Autodesk Fusion 360 part; units mm, degrees
(part 2 of 3)
  spline S228 degree 3 poles (-3.1149, 116.9539) (-3.0452, 117.0404) (-2.9015, 117.2184) (-2.6994, 117.3259) (-2.5954, 117.3812) knots 0 0 0 0 0.032959 0.067885 0.067885 0.067885 0.067885
  spline S229 degree 3 poles (-3.3935, 116.2276) (-3.362, 116.3667) (-3.304, 116.6225) (-3.1742, 116.8501) (-3.1149, 116.9539) knots 0 0 0 0 0.042495 0.07817 0.07817 0.07817 0.07817
  line L121 (-3.3935, 116.2276) -> (-2.5083, 116.0772)
  spline S230 degree 3 poles (-2.2963, 116.5763) (-2.3491, 116.5089) (-2.4641, 116.3621) (-2.4927, 116.1772) (-2.5083, 116.0772) knots 0 0 0 0 0.025264 0.055024 0.055024 0.055024 0.055024
  spline S231 degree 3 poles (-1.8759, 116.7471) (-1.9549, 116.7401) (-2.1125, 116.726) (-2.2351, 116.6261) (-2.2963, 116.5763) knots 0 0 0 0 0.023212 0.046318 0.046318 0.046318 0.046318
  spline S232 degree 3 poles (-1.476, 116.5968) (-1.532, 116.6406) (-1.6492, 116.7324) (-1.7981, 116.7421) (-1.8759, 116.7471) knots 0 0 0 0 0.020834 0.04362 0.04362 0.04362 0.04362
  spline S233 degree 3 poles (-1.3256, 116.1934) (-1.3306, 116.2721) (-1.34, 116.4222) (-1.4322, 116.5405) (-1.476, 116.5968) knots 0 0 0 0 0.023038 0.043945 0.043945 0.043945 0.043945
  spline S234 degree 3 poles (-1.5307, 115.7166) (-1.4709, 115.7825) (-1.3482, 115.9178) (-1.3333, 116.1) (-1.3256, 116.1934) knots 0 0 0 0 0.025943 0.053218 0.053218 0.053218 0.053218
  spline S235 degree 3 poles (-2.1254, 115.5474) (-2.0075, 115.5485) (-1.7927, 115.5505) (-1.6121, 115.665) (-1.5307, 115.7166) knots 0 0 0 0 0.034551 0.062931 0.062931 0.062931 0.062931
  line L122 (-2.1254, 115.5474) -> (-2.2314, 114.7647)
  spline S236 degree 3 poles (-1.7905, 114.8365) (-1.8583, 114.8326) (-2.0077, 114.8239) (-2.1524, 114.7856) (-2.2314, 114.7647) knots 0 0 0 0 0.020331 0.044771 0.044771 0.044771 0.044771
  spline S237 degree 3 poles (-1.3154, 114.6246) (-1.3835, 114.6864) (-1.5188, 114.8091) (-1.7004, 114.8274) (-1.7905, 114.8365) knots 0 0 0 0 0.026832 0.05326 0.05326 0.05326 0.05326
  spline S238 degree 3 poles (-1.1206, 114.0504) (-1.1264, 114.1623) (-1.1374, 114.3727) (-1.2586, 114.5443) (-1.3154, 114.6246) knots 0 0 0 0 0.032834 0.061749 0.061749 0.061749 0.061749
  spline S239 degree 3 poles (-1.3239, 113.442) (-1.2647, 113.5273) (-1.1381, 113.7097) (-1.1267, 113.9321) (-1.1206, 114.0504) knots 0 0 0 0 0.030567 0.065292 0.065292 0.065292 0.065292
  spline S240 degree 3 poles (-1.8247, 113.2164) (-1.7293, 113.226) (-1.5373, 113.2454) (-1.3953, 113.3762) (-1.3239, 113.442) knots 0 0 0 0 0.027961 0.056262 0.056262 0.056262 0.056262
  spline S241 degree 3 poles (-2.2963, 113.4044) (-2.2277, 113.3495) (-2.0895, 113.2392) (-1.9133, 113.224) (-1.8247, 113.2164) knots 0 0 0 0 0.025738 0.0518 0.0518 0.0518 0.0518
  spline S242 degree 3 poles (-2.5356, 113.9478) (-2.5173, 113.8392) (-2.4833, 113.6372) (-2.3554, 113.4779) (-2.2963, 113.4044) knots 0 0 0 0 0.032415 0.060264 0.060264 0.060264 0.060264
  line L123 (-2.5356, 113.9478) -> (-3.4653, 113.835)
  spline S243 degree 3 poles (-2.9458, 112.8114) (-3.0795, 112.9538) (-3.3522, 113.244) (-3.4271, 113.6356) (-3.4653, 113.835) knots 0 0 0 0 0.057366 0.116928 0.116928 0.116928 0.116928
  line L124 (-5.3383, 113.2266) -> (-5.3383, 114.5289)
  line L125 (-5.3383, 114.5289) -> (-4.0224, 114.5289)
  line L126 (-4.0224, 114.5289) -> (-4.0224, 115.4278)
  line L127 (-4.0224, 115.4278) -> (-5.3383, 115.4278)
  line L128 (-5.3383, 115.4278) -> (-5.3383, 116.7301)
  line L129 (-5.3383, 116.7301) -> (-6.2133, 116.7301)
  line L130 (-6.2133, 116.7301) -> (-6.2133, 115.4278)
  line L131 (-6.2133, 115.4278) -> (-7.5258, 115.4278)
  line L132 (-7.5258, 115.4278) -> (-7.5258, 114.5289)
  line L133 (-7.5258, 114.5289) -> (-6.2133, 114.5289)
  line L134 (-6.2133, 114.5289) -> (-6.2133, 113.2266)
  line L135 (-6.2133, 113.2266) -> (-5.3383, 113.2266)
  line L136 (20.9668, 130.42) -> (22.8707, 130.42)
  spline S244 degree 3 poles (23.7662, 130.526) (23.6363, 130.4952) (23.3421, 130.4254) (23.0396, 130.4219) (22.8707, 130.42) knots 0 0 0 0 0.039934 0.090419 0.090419 0.090419 0.090419
  spline S245 degree 3 poles (24.4771, 130.9259) (24.3774, 130.8438) (24.1645, 130.6685) (23.9045, 130.5754) (23.7662, 130.526) knots 0 0 0 0 0.038436 0.082116 0.082116 0.082116 0.082116
  spline S246 degree 3 poles (25.0137, 131.8111) (24.9472, 131.6403) (24.82, 131.3136) (24.5879, 131.0511) (24.4771, 130.9259) knots 0 0 0 0 0.054482 0.104246 0.104246 0.104246 0.104246
  spline S247 degree 3 poles (25.1675, 132.8775) (25.1631, 132.6843) (25.1547, 132.3224) (25.0585, 131.9737) (25.0137, 131.8111) knots 0 0 0 0 0.057721 0.108107 0.108107 0.108107 0.108107
  spline S248 degree 3 poles (25.0035, 134.0618) (25.0512, 133.8841) (25.1554, 133.4965) (25.1633, 133.0949) (25.1675, 132.8775) knots 0 0 0 0 0.055013 0.119956 0.119956 0.119956 0.119956
  spline S249 degree 3 poles (24.525, 134.8736) (24.6242, 134.7548) (24.8282, 134.5107) (24.944, 134.2141) (25.0035, 134.0618) knots 0 0 0 0 0.046108 0.094787 0.094787 0.094787 0.094787
  spline S250 degree 3 poles (23.7696, 135.335) (23.9112, 135.2834) (24.194, 135.1804) (24.4148, 134.9758) (24.525, 134.8736) knots 0 0 0 0 0.044725 0.089312 0.089312 0.089312 0.089312
  spline S251 degree 3 poles (22.816, 135.4307) (23.0005, 135.4297) (23.3217, 135.428) (23.6358, 135.3628) (23.7696, 135.335) knots 0 0 0 0 0.055167 0.096048 0.096048 0.096048 0.096048
  line L137 (22.816, 135.4307) -> (20.9668, 135.4307)
  line L138 (20.9668, 135.4307) -> (20.9668, 130.42)
  spline S252 degree 3 poles (23.2637, 134.5352) (23.1593, 134.549) (22.8839, 134.5853) (22.6058, 134.5839) (22.4332, 134.5831) knots 0 0 0 0 0.031565 0.083275 0.083275 0.083275 0.083275
  spline S253 degree 3 poles (23.732, 134.2994) (23.6648, 134.3531) (23.5254, 134.4645) (23.353, 134.5111) (23.2637, 134.5352) knots 0 0 0 0 0.02553 0.052932 0.052932 0.052932 0.052932
  spline S254 degree 3 poles (24.0191, 133.814) (23.9838, 133.9098) (23.9176, 134.0893) (23.7911, 134.2325) (23.732, 134.2994) knots 0 0 0 0 0.030297 0.056827 0.056827 0.056827 0.056827
  spline S255 degree 3 poles (24.1216, 132.922) (24.1204, 133.0941) (24.1182, 133.3954) (24.0488, 133.6884) (24.0191, 133.814) knots 0 0 0 0 0.051419 0.090046 0.090046 0.090046 0.090046
  spline S256 degree 3 poles (24.0191, 132.0042) (24.0489, 132.1363) (24.1169, 132.4381) (24.1199, 132.7478) (24.1216, 132.922) knots 0 0 0 0 0.040513 0.092572 0.092572 0.092572 0.092572
  spline S257 degree 3 poles (23.7542, 131.5206) (23.8074, 131.5831) (23.9287, 131.7255) (23.9866, 131.904) (24.0191, 132.0042) knots 0 0 0 0 0.024396 0.055616 0.055616 0.055616 0.055616
  spline S258 degree 3 poles (23.3458, 131.3121) (23.4232, 131.3352) (23.5723, 131.3796) (23.6951, 131.4748) (23.7542, 131.5206) knots 0 0 0 0 0.023993 0.046213 0.046213 0.046213 0.046213
  spline S259 degree 3 poles (22.7339, 131.2642) (22.8559, 131.2642) (23.0613, 131.2642) (23.2636, 131.2983) (23.3458, 131.3121) knots 0 0 0 0 0.036506 0.061461 0.061461 0.061461 0.061461
  line L139 (22.7339, 131.2642) -> (21.9786, 131.2642)
  line L140 (21.9786, 131.2642) -> (21.9786, 134.5831)
  line L141 (21.9786, 134.5831) -> (22.4332, 134.5831)
  line L142 (26.9517, 130.42) -> (26.9517, 134.3643)
  line L143 (26.9517, 134.3643) -> (27.9429, 130.42)
  line L144 (27.9429, 130.42) -> (28.917, 130.42)
  line L145 (28.917, 130.42) -> (29.9117, 134.3643)
  line L146 (29.9117, 134.3643) -> (29.9117, 130.42)
  line L147 (29.9117, 130.42) -> (30.8516, 130.42)
  line L148 (30.8516, 130.42) -> (30.8516, 135.4307)
  line L149 (30.8516, 135.4307) -> (29.334, 135.4307)
  line L150 (29.334, 135.4307) -> (28.4351, 132.0128)
  line L151 (28.4351, 132.0128) -> (27.5259, 135.4307)
  line L152 (27.5259, 135.4307) -> (26.0118, 135.4307)
  line L153 (26.0118, 135.4307) -> (26.0118, 130.42)
  line L154 (26.0118, 130.42) -> (26.9517, 130.42)
  line L155 (32.7828, 130.42) -> (32.7828, 134.3643)
  line L156 (32.7828, 134.3643) -> (33.774, 130.42)
  line L157 (33.774, 130.42) -> (34.7481, 130.42)
  line L158 (34.7481, 130.42) -> (35.7427, 134.3643)
  line L159 (35.7427, 134.3643) -> (35.7427, 130.42)
  line L160 (35.7427, 130.42) -> (36.6827, 130.42)
  line L161 (36.6827, 130.42) -> (36.6827, 135.4307)
  line L162 (36.6827, 135.4307) -> (35.1651, 135.4307)
  line L163 (35.1651, 135.4307) -> (34.2662, 132.0128)
  line L164 (34.2662, 132.0128) -> (33.357, 135.4307)
  line L165 (33.357, 135.4307) -> (31.8428, 135.4307)
  line L166 (31.8428, 135.4307) -> (31.8428, 130.42)
  line L167 (31.8428, 130.42) -> (32.7828, 130.42)
  line L168 (39.9332, 135.4513) -> (39.1539, 135.4513)
  spline S260 degree 3 poles (38.5489, 134.6497) (38.6832, 134.766) (38.9423, 134.9903) (39.0851, 135.3014) (39.1539, 135.4513) knots 0 0 0 0 0.052597 0.101463 0.101463 0.101463 0.101463
  spline S261 degree 3 poles (37.732, 134.1832) (37.8654, 134.2377) (38.1579, 134.3572) (38.4112, 134.5467) (38.5489, 134.6497) knots 0 0 0 0 0.043078 0.094413 0.094413 0.094413 0.094413
  line L169 (37.732, 134.1832) -> (37.732, 133.3116)
  spline S262 degree 3 poles (38.9727, 134.0396) (38.7881, 133.8858) (38.4148, 133.5747) (37.9613, 133.4) (37.732, 133.3116) knots 0 0 0 0 0.071555 0.144721 0.144721 0.144721 0.144721
  line L170 (38.9727, 134.0396) -> (38.9727, 130.42)
  line L171 (38.9727, 130.42) -> (39.9332, 130.42)
  line L172 (39.9332, 130.42) -> (39.9332, 135.4513)
  line L173 (20.5738, 112.42) -> (22.4776, 112.42)
  spline S263 degree 3 poles (23.3731, 112.526) (23.2432, 112.4952) (22.9491, 112.4254) (22.6465, 112.4219) (22.4776, 112.42) knots 0 0 0 0 0.039934 0.090419 0.090419 0.090419 0.090419
  spline S264 degree 3 poles (24.084, 112.9259) (23.9844, 112.8438) (23.7714, 112.6685) (23.5114, 112.5754) (23.3731, 112.526) knots 0 0 0 0 0.038436 0.082116 0.082116 0.082116 0.082116
  spline S265 degree 3 poles (24.6207, 113.8111) (24.5541, 113.6403) (24.4269, 113.3136) (24.1948, 113.0511) (24.084, 112.9259) knots 0 0 0 0 0.054482 0.104246 0.104246 0.104246 0.104246
  spline S266 degree 3 poles (24.7745, 114.8775) (24.77, 114.6843) (24.7616, 114.3224) (24.6655, 113.9737) (24.6207, 113.8111) knots 0 0 0 0 0.057721 0.108107 0.108107 0.108107 0.108107
  spline S267 degree 3 poles (24.6104, 116.0618) (24.6582, 115.8841) (24.7623, 115.4965) (24.7702, 115.0949) (24.7745, 114.8775) knots 0 0 0 0 0.055013 0.119956 0.119956 0.119956 0.119956
  spline S268 degree 3 poles (24.1319, 116.8736) (24.2311, 116.7548) (24.4352, 116.5107) (24.5509, 116.2141) (24.6104, 116.0618) knots 0 0 0 0 0.046108 0.094787 0.094787 0.094787 0.094787
  spline S269 degree 3 poles (23.3765, 117.335) (23.5181, 117.2834) (23.8009, 117.1804) (24.0217, 116.9758) (24.1319, 116.8736) knots 0 0 0 0 0.044725 0.089312 0.089312 0.089312 0.089312
  spline S270 degree 3 poles (22.4229, 117.4307) (22.6074, 117.4297) (22.9286, 117.428) (23.2428, 117.3628) (23.3765, 117.335) knots 0 0 0 0 0.055167 0.096048 0.096048 0.096048 0.096048
  line L174 (22.4229, 117.4307) -> (20.5738, 117.4307)
  line L175 (20.5738, 117.4307) -> (20.5738, 112.42)
  spline S271 degree 3 poles (22.8707, 116.5352) (22.7662, 116.549) (22.4908, 116.5853) (22.2127, 116.5839) (22.0401, 116.5831) knots 0 0 0 0 0.031565 0.083275 0.083275 0.083275 0.083275
  spline S272 degree 3 poles (23.3389, 116.2994) (23.2717, 116.3531) (23.1323, 116.4645) (22.9599, 116.5111) (22.8707, 116.5352) knots 0 0 0 0 0.02553 0.052932 0.052932 0.052932 0.052932
  spline S273 degree 3 poles (23.626, 115.814) (23.5907, 115.9098) (23.5245, 116.0893) (23.398, 116.2325) (23.3389, 116.2994) knots 0 0 0 0 0.030297 0.056827 0.056827 0.056827 0.056827
  spline S274 degree 3 poles (23.7286, 114.922) (23.7273, 115.0941) (23.7251, 115.3954) (23.6558, 115.6884) (23.626, 115.814) knots 0 0 0 0 0.051419 0.090046 0.090046 0.090046 0.090046
  spline S275 degree 3 poles (23.626, 114.0042) (23.6558, 114.1363) (23.7239, 114.4381) (23.7269, 114.7478) (23.7286, 114.922) knots 0 0 0 0 0.040513 0.092572 0.092572 0.092572 0.092572
  spline S276 degree 3 poles (23.3611, 113.5206) (23.4143, 113.5831) (23.5356, 113.7255) (23.5935, 113.904) (23.626, 114.0042) knots 0 0 0 0 0.024396 0.055616 0.055616 0.055616 0.055616
  spline S277 degree 3 poles (22.9527, 113.3121) (23.0301, 113.3352) (23.1792, 113.3796) (23.3021, 113.4748) (23.3611, 113.5206) knots 0 0 0 0 0.023993 0.046213 0.046213 0.046213 0.046213
  spline S278 degree 3 poles (22.3409, 113.2642) (22.4628, 113.2642) (22.6682, 113.2642) (22.8705, 113.2983) (22.9527, 113.3121) knots 0 0 0 0 0.036506 0.061461 0.061461 0.061461 0.061461
  line L176 (22.3409, 113.2642) -> (21.5855, 113.2642)
  line L177 (21.5855, 113.2642) -> (21.5855, 116.5831)
  line L178 (21.5855, 116.5831) -> (22.0401, 116.5831)
  line L179 (26.5586, 112.42) -> (26.5586, 116.3643)
  line L180 (26.5586, 116.3643) -> (27.5499, 112.42)
  line L181 (27.5499, 112.42) -> (28.524, 112.42)
  line L182 (28.524, 112.42) -> (29.5186, 116.3643)
  line L183 (29.5186, 116.3643) -> (29.5186, 112.42)
  line L184 (29.5186, 112.42) -> (30.4585, 112.42)
  line L185 (30.4585, 112.42) -> (30.4585, 117.4307)
  line L186 (30.4585, 117.4307) -> (28.941, 117.4307)
  line L187 (28.941, 117.4307) -> (28.042, 114.0128)
  line L188 (28.042, 114.0128) -> (27.1329, 117.4307)
  line L189 (27.1329, 117.4307) -> (25.6187, 117.4307)
  line L190 (25.6187, 117.4307) -> (25.6187, 112.42)
  line L191 (25.6187, 112.42) -> (26.5586, 112.42)
  line L192 (32.3897, 112.42) -> (32.3897, 116.3643)
  line L193 (32.3897, 116.3643) -> (33.3809, 112.42)
  line L194 (33.3809, 112.42) -> (34.355, 112.42)
  line L195 (34.355, 112.42) -> (35.3497, 116.3643)
  line L196 (35.3497, 116.3643) -> (35.3497, 112.42)
  line L197 (35.3497, 112.42) -> (36.2896, 112.42)
  line L198 (36.2896, 112.42) -> (36.2896, 117.4307)
  line L199 (36.2896, 117.4307) -> (34.772, 117.4307)
  line L200 (34.772, 117.4307) -> (33.8731, 114.0128)
  line L201 (33.8731, 114.0128) -> (32.9639, 117.4307)
  line L202 (32.9639, 117.4307) -> (31.4498, 117.4307)
  line L203 (31.4498, 117.4307) -> (31.4498, 112.42)
  line L204 (31.4498, 112.42) -> (32.3897, 112.42)
  spline S279 degree 3 poles (38.6155, 113.5787) (38.5777, 113.5346) (38.5056, 113.4505) (38.4469, 113.3567) (38.419, 113.3121) knots 0 0 0 0 0.017402 0.033163 0.033163 0.033163 0.033163
  spline S280 degree 3 poles (39.1915, 114.1324) (39.0662, 114.0183) (38.8693, 113.8388) (38.6833, 113.6481) (38.6155, 113.5787) knots 0 0 0 0 0.050814 0.079907 0.079907 0.079907 0.079907
  spline S281 degree 3 poles (39.8204, 114.7716) (39.7402, 114.68) (39.543, 114.4549) (39.3224, 114.2525) (39.1915, 114.1324) knots 0 0 0 0 0.036482 0.089726 0.089726 0.089726 0.089726
  spline S282 degree 3 poles (40.2049, 115.4124) (40.156, 115.306) (40.0513, 115.0785) (39.9006, 114.8782) (39.8204, 114.7716) knots 0 0 0 0 0.035023 0.074928 0.074928 0.074928 0.074928
  spline S283 degree 3 poles (40.3262, 116.0567) (40.3213, 115.9456) (40.3116, 115.7251) (40.2403, 115.5162) (40.2049, 115.4124) knots 0 0 0 0 0.033165 0.06586 0.06586 0.06586 0.06586
  spline S284 degree 3 poles (39.9024, 117.0513) (40.026, 116.9094) (40.2747, 116.6237) (40.309, 116.2465) (40.3262, 116.0567) knots 0 0 0 0 0.054981 0.110602 0.110602 0.110602 0.110602
  spline S285 degree 3 poles (38.7369, 117.4513) (38.9653, 117.4395) (39.3937, 117.4175) (39.7405, 117.1678) (39.9024, 117.0513) knots 0 0 0 0 0.066974 0.125562 0.125562 0.125562 0.125562
  spline S286 degree 3 poles (37.6089, 117.106) (37.7736, 117.2067) (38.1193, 117.4179) (38.5246, 117.4398) (38.7369, 117.4513) knots 0 0 0 0 0.056979 0.119613 0.119613 0.119613 0.119613
  spline S287 degree 3 poles (37.0723, 115.9679) (37.1077, 116.2065) (37.1724, 116.6426) (37.4729, 116.9616) (37.6089, 117.106) knots 0 0 0 0 0.070363 0.128535 0.128535 0.128535 0.128535
  line L205 (37.0723, 115.9679) -> (38.0293, 115.8721)
  spline S288 degree 3 poles (38.2344, 116.4737) (38.1812, 116.3958) (38.0579, 116.2155) (38.0397, 115.9965) (38.0293, 115.8721) knots 0 0 0 0 0.027875 0.064515 0.064515 0.064515 0.064515
  spline S289 degree 3 poles (38.7129, 116.6549) (38.6194, 116.6489) (38.4408, 116.6374) (38.301, 116.5265) (38.2344, 116.4737) knots 0 0 0 0 0.027379 0.052265 0.052265 0.052265 0.052265
  spline S290 degree 3 poles (39.1897, 116.4823) (39.1239, 116.5325) (38.9837, 116.6397) (38.8068, 116.6496) (38.7129, 116.6549) knots 0 0 0 0 0.024288 0.051759 0.051759 0.051759 0.051759
  spline S291 degree 3 poles (39.3624, 115.9884) (39.3576, 116.0866) (39.3489, 116.2692) (39.24, 116.4149) (39.1897, 116.4823) knots 0 0 0 0 0.028738 0.053388 0.053388 0.053388 0.053388
  spline S292 degree 3 poles (39.1641, 115.4005) (39.2219, 115.4963) (39.3314, 115.678) (39.3524, 115.8888) (39.3624, 115.9884) knots 0 0 0 0 0.033093 0.062734 0.062734 0.062734 0.062734
  spline S293 degree 3 poles (38.3677, 114.5802) (38.5471, 114.7449) (38.8284, 115.0032) (39.0748, 115.2948) (39.1641, 115.4005) knots 0 0 0 0 0.072938 0.114424 0.114424 0.114424 0.114424
  spline S294 degree 3 poles (37.2876, 113.3787) (37.4189, 113.5582) (37.7381, 113.9945) (38.1344, 114.3631) (38.3677, 114.5802) knots 0 0 0 0 0.066554 0.16187 0.16187 0.16187 0.16187
  spline S295 degree 3 poles (36.9595, 112.42) (36.9873, 112.5872) (37.0435, 112.9249) (37.2057, 113.2264) (37.2876, 113.3787) knots 0 0 0 0 0.050461 0.101951 0.101951 0.101951 0.101951
  line L206 (36.9595, 112.42) -> (40.3262, 112.42)
  line L207 (40.3262, 112.42) -> (40.3262, 113.3121)
  line L208 (40.3262, 113.3121) -> (38.419, 113.3121)
  line L209 (24.0248, 96.3377) -> (24.0248, 95.702)
  spline S296 degree 3 poles (23.4762, 95.3995) (23.5772, 95.4419) (23.7708, 95.5233) (23.9426, 95.6441) (24.0248, 95.702) knots 0 0 0 0 0.032744 0.062808 0.062808 0.062808 0.062808
  spline S297 degree 3 poles (22.8388, 95.2747) (22.9458, 95.2803) (23.1641, 95.2917) (23.3708, 95.3631) (23.4762, 95.3995) knots 0 0 0 0 0.031982 0.065241 0.065241 0.065241 0.065241
  spline S298 degree 3 poles (21.7997, 95.7208) (21.9443, 95.5907) (22.2397, 95.3249) (22.6363, 95.2917) (22.8388, 95.2747) knots 0 0 0 0 0.056717 0.115883 0.115883 0.115883 0.115883
  spline S299 degree 3 poles (21.4032, 97.0589) (21.4112, 96.7908) (21.4256, 96.3072) (21.6844, 95.9015) (21.7997, 95.7208) knots 0 0 0 0 0.078685 0.141874 0.141874 0.141874 0.141874
  spline S300 degree 3 poles (21.7946, 98.3065) (21.6807, 98.1378) (21.4277, 97.763) (21.4119, 97.3088) (21.4032, 97.0589) knots 0 0 0 0 0.059895 0.133098 0.133098 0.133098 0.133098
  spline S301 degree 3 poles (22.849, 98.7269) (22.6422, 98.7124) (22.2448, 98.6846) (21.9405, 98.429) (21.7946, 98.3065) knots 0 0 0 0 0.060436 0.116147 0.116147 0.116147 0.116147
  spline S302 degree 3 poles (23.5787, 98.5133) (23.4719, 98.5755) (23.2468, 98.7067) (22.986, 98.72) (22.849, 98.7269) knots 0 0 0 0 0.036554 0.077026 0.077026 0.077026 0.077026
  spline S303 degree 3 poles (23.9769, 97.9305) (23.9347, 98.0465) (23.8514, 98.2748) (23.6687, 98.4346) (23.5787, 98.5133) knots 0 0 0 0 0.036378 0.071607 0.071607 0.071607 0.071607
  line L210 (23.9769, 97.9305) -> (24.9818, 98.1185)
  spline S304 degree 3 poles (24.3068, 99.2003) (24.4666, 99.055) (24.793, 98.7583) (24.918, 98.3347) (24.9818, 98.1185) knots 0 0 0 0 0.063491 0.129715 0.129715 0.129715 0.129715
  spline S305 degree 3 poles (22.849, 99.5916) (23.1327, 99.5825) (23.651, 99.5657) (24.1024, 99.3142) (24.3068, 99.2003) knots 0 0 0 0 0.083673 0.152883 0.152883 0.152883 0.152883
  spline S306 degree 3 poles (21.6493, 99.3421) (21.8274, 99.4148) (22.2113, 99.5715) (22.6264, 99.5846) (22.849, 99.5916) knots 0 0 0 0 0.057235 0.123411 0.123411 0.123411 0.123411
  spline S307 degree 3 poles (20.6888, 98.409) (20.8117, 98.6004) (21.0592, 98.986) (21.4516, 99.2228) (21.6493, 99.3421) knots 0 0 0 0 0.067249 0.13551 0.13551 0.13551 0.13551
  spline S308 degree 3 poles (20.3607, 97.0179) (20.3725, 97.268) (20.3954, 97.7525) (20.5932, 98.195) (20.6888, 98.409) knots 0 0 0 0 0.074367 0.144055 0.144055 0.144055 0.144055
  spline S309 degree 3 poles (20.6547, 95.6832) (20.5689, 95.894) (20.3948, 96.322) (20.3722, 96.7836) (20.3607, 97.0179) knots 0 0 0 0 0.067732 0.137548 0.137548 0.137548 0.137548
  spline S310 degree 3 poles (21.5331, 94.7398) (21.3502, 94.862) (20.9831, 95.1071) (20.7644, 95.4907) (20.6547, 95.6832) knots 0 0 0 0 0.065007 0.130489 0.130489 0.130489 0.130489
  spline S311 degree 3 poles (22.9037, 94.41) (22.6545, 94.4213) (22.1759, 94.443) (21.7413, 94.6437) (21.5331, 94.7398) knots 0 0 0 0 0.074032 0.14217 0.14217 0.14217 0.14217
  spline S312 degree 3 poles (24.1256, 94.6441) (23.9251, 94.5758) (23.5286, 94.4408) (23.1104, 94.4202) (22.9037, 94.41) knots 0 0 0 0 0.0632 0.124959 0.124959 0.124959 0.124959
  spline S313 degree 3 poles (25.0468, 95.1859) (24.9207, 95.0833) (24.6416, 94.8563) (24.3083, 94.7193) (24.1256, 94.6441) knots 0 0 0 0 0.048493 0.107374 0.107374 0.107374 0.107374
  line L211 (25.0468, 95.1859) -> (25.0468, 97.182)
  line L212 (25.0468, 97.182) -> (22.8661, 97.182)
  line L213 (22.8661, 97.182) -> (22.8661, 96.3377)
  line L214 (22.8661, 96.3377) -> (24.0248, 96.3377)
  line L215 (26.9301, 94.4954) -> (26.9301, 97.763)
  line L216 (26.9301, 97.763) -> (28.9501, 94.4954)
  line L217 (28.9501, 94.4954) -> (29.9652, 94.4954)
  line L218 (29.9652, 94.4954) -> (29.9652, 99.5062)
  line L219 (29.9652, 99.5062) -> (29.0253, 99.5062)
  line L220 (29.0253, 99.5062) -> (29.0253, 96.16)
  line L221 (29.0253, 96.16) -> (26.9745, 99.5062)
  line L222 (26.9745, 99.5062) -> (25.9901, 99.5062)
  line L223 (25.9901, 99.5062) -> (25.9901, 94.4954)
  line L224 (25.9901, 94.4954) -> (26.9301, 94.4954)
  line L225 (31.0316, 94.4954) -> (32.9354, 94.4954)
  spline S314 degree 3 poles (33.8309, 94.6014) (33.701, 94.5706) (33.4069, 94.5009) (33.1044, 94.4974) (32.9354, 94.4954) knots 0 0 0 0 0.039934 0.090419 0.090419 0.090419 0.090419
  spline S315 degree 3 poles (34.5419, 95.0013) (34.4422, 94.9193) (34.2293, 94.7439) (33.9693, 94.6509) (33.8309, 94.6014) knots 0 0 0 0 0.038436 0.082116 0.082116 0.082116 0.082116
  spline S316 degree 3 poles (35.0785, 95.8866) (35.012, 95.7158) (34.8847, 95.389) (34.6527, 95.1266) (34.5419, 95.0013) knots 0 0 0 0 0.054482 0.104246 0.104246 0.104246 0.104246
  spline S317 degree 3 poles (35.2323, 96.953) (35.2278, 96.7597) (35.2194, 96.3978) (35.1233, 96.0491) (35.0785, 95.8866) knots 0 0 0 0 0.057721 0.108107 0.108107 0.108107 0.108107
  spline S318 degree 3 poles (35.0682, 98.1373) (35.116, 97.9595) (35.2202, 97.572) (35.228, 97.1704) (35.2323, 96.953) knots 0 0 0 0 0.055013 0.119956 0.119956 0.119956 0.119956
  spline S319 degree 3 poles (34.5897, 98.9491) (34.689, 98.8303) (34.893, 98.5861) (35.0088, 98.2896) (35.0682, 98.1373) knots 0 0 0 0 0.046108 0.094787 0.094787 0.094787 0.094787
  spline S320 degree 3 poles (33.8344, 99.4105) (33.976, 99.3589) (34.2588, 99.2558) (34.4795, 99.0512) (34.5897, 98.9491) knots 0 0 0 0 0.044725 0.089312 0.089312 0.089312 0.089312
  spline S321 degree 3 poles (32.8807, 99.5062) (33.0652, 99.5052) (33.3864, 99.5035) (33.7006, 99.4382) (33.8344, 99.4105) knots 0 0 0 0 0.055167 0.096048 0.096048 0.096048 0.096048
  line L226 (32.8807, 99.5062) -> (31.0316, 99.5062)
  line L227 (31.0316, 99.5062) -> (31.0316, 94.4954)
  spline S322 degree 3 poles (33.3285, 98.6107) (33.2241, 98.6245) (32.9486, 98.6608) (32.6706, 98.6594) (32.4979, 98.6585) knots 0 0 0 0 0.031564 0.083275 0.083275 0.083275 0.083275
  spline S323 degree 3 poles (33.7968, 98.3748) (33.7295, 98.4286) (33.5902, 98.54) (33.4178, 98.5866) (33.3285, 98.6107) knots 0 0 0 0 0.02553 0.052932 0.052932 0.052932 0.052932
  spline S324 degree 3 poles (34.0839, 97.8895) (34.0486, 97.9852) (33.9824, 98.1648) (33.8558, 98.308) (33.7968, 98.3748) knots 0 0 0 0 0.030297 0.056827 0.056827 0.056827 0.056827
  spline S325 degree 3 poles (34.1864, 96.9974) (34.1852, 97.1695) (34.183, 97.4709) (34.1136, 97.7638) (34.0839, 97.8895) knots 0 0 0 0 0.051419 0.090046 0.090046 0.090046 0.090046
  spline S326 degree 3 poles (34.0839, 96.0797) (34.1137, 96.2118) (34.1817, 96.5136) (34.1847, 96.8233) (34.1864, 96.9974) knots 0 0 0 0 0.040513 0.092572 0.092572 0.092572 0.092572
  spline S327 degree 3 poles (33.819, 95.596) (33.8722, 95.6585) (33.9934, 95.801) (34.0514, 95.9795) (34.0839, 96.0797) knots 0 0 0 0 0.024396 0.055616 0.055616 0.055616 0.055616
  spline S328 degree 3 poles (33.4105, 95.3875) (33.4879, 95.4106) (33.637, 95.455) (33.7599, 95.5503) (33.819, 95.596) knots 0 0 0 0 0.023993 0.046213 0.046213 0.046213 0.046213
  spline S329 degree 3 poles (32.7987, 95.3397) (32.9207, 95.3397) (33.126, 95.3396) (33.3284, 95.3737) (33.4105, 95.3875) knots 0 0 0 0 0.036506 0.061461 0.061461 0.061461 0.061461
  line L228 (32.7987, 95.3397) -> (32.0433, 95.3397)
  line L229 (32.0433, 95.3397) -> (32.0433, 98.6585)
  line L230 (32.0433, 98.6585) -> (32.4979, 98.6585)
  line L231 (-13.5136, 96.3377) -> (-13.5136, 95.702)
  spline S330 degree 3 poles (-14.0622, 95.3995) (-13.9612, 95.4419) (-13.7675, 95.5233) (-13.5958, 95.6441) (-13.5136, 95.702) knots 0 0 0 0 0.032744 0.062808 0.062808 0.062808 0.062808
  spline S331 degree 3 poles (-14.6996, 95.2747) (-14.5926, 95.2803) (-14.3742, 95.2917) (-14.1675, 95.3631) (-14.0622, 95.3995) knots 0 0 0 0 0.031982 0.065241 0.065241 0.065241 0.065241
  spline S332 degree 3 poles (-15.7387, 95.7208) (-15.5941, 95.5907) (-15.2987, 95.3249) (-14.9021, 95.2917) (-14.6996, 95.2747) knots 0 0 0 0 0.056717 0.115883 0.115883 0.115883 0.115883
  spline S333 degree 3 poles (-16.1352, 97.0589) (-16.1272, 96.7908) (-16.1128, 96.3072) (-15.854, 95.9015) (-15.7387, 95.7208) knots 0 0 0 0 0.078685 0.141874 0.141874 0.141874 0.141874
  spline S334 degree 3 poles (-15.7438, 98.3065) (-15.8577, 98.1378) (-16.1106, 97.763) (-16.1265, 97.3088) (-16.1352, 97.0589) knots 0 0 0 0 0.059895 0.133098 0.133098 0.133098 0.133098
  spline S335 degree 3 poles (-14.6894, 98.7269) (-14.8961, 98.7124) (-15.2936, 98.6846) (-15.5978, 98.429) (-15.7438, 98.3065) knots 0 0 0 0 0.060436 0.116147 0.116147 0.116147 0.116147
  spline S336 degree 3 poles (-13.9596, 98.5133) (-14.0665, 98.5755) (-14.2916, 98.7067) (-14.5524, 98.72) (-14.6894, 98.7269) knots 0 0 0 0 0.036554 0.077026 0.077026 0.077026 0.077026
  spline S337 degree 3 poles (-13.5614, 97.9305) (-13.6037, 98.0465) (-13.6869, 98.2748) (-13.8697, 98.4346) (-13.9596, 98.5133) knots 0 0 0 0 0.036378 0.071607 0.071607 0.071607 0.071607
  line L232 (-13.5614, 97.9305) -> (-12.5565, 98.1185)
  spline S338 degree 3 poles (-13.2316, 99.2003) (-13.0718, 99.055) (-12.7454, 98.7583) (-12.6204, 98.3347) (-12.5565, 98.1185) knots 0 0 0 0 0.063491 0.129715 0.129715 0.129715 0.129715
  spline S339 degree 3 poles (-14.6894, 99.5916) (-14.4057, 99.5825) (-13.8874, 99.5657) (-13.4359, 99.3142) (-13.2316, 99.2003) knots 0 0 0 0 0.083673 0.152883 0.152883 0.152883 0.152883
  spline S340 degree 3 poles (-15.8891, 99.3421) (-15.711, 99.4148) (-15.3271, 99.5715) (-14.9119, 99.5846) (-14.6894, 99.5916) knots 0 0 0 0 0.057235 0.123411 0.123411 0.123411 0.123411
  spline S341 degree 3 poles (-16.8495, 98.409) (-16.7267, 98.6004) (-16.4792, 98.986) (-16.0867, 99.2228) (-15.8891, 99.3421) knots 0 0 0 0 0.067249 0.13551 0.13551 0.13551 0.13551
  spline S342 degree 3 poles (-17.1776, 97.0179) (-17.1658, 97.268) (-17.143, 97.7525) (-16.9452, 98.195) (-16.8495, 98.409) knots 0 0 0 0 0.074367 0.144055 0.144055 0.144055 0.144055
  spline S343 degree 3 poles (-16.8837, 95.6832) (-16.9694, 95.894) (-17.1435, 96.322) (-17.1662, 96.7836) (-17.1776, 97.0179) knots 0 0 0 0 0.067732 0.137548 0.137548 0.137548 0.137548
  spline S344 degree 3 poles (-16.0053, 94.7398) (-16.1882, 94.862) (-16.5553, 95.1071) (-16.774, 95.4907) (-16.8837, 95.6832) knots 0 0 0 0 0.065007 0.130489 0.130489 0.130489 0.130489
  spline S345 degree 3 poles (-14.6347, 94.41) (-14.8839, 94.4213) (-15.3625, 94.443) (-15.797, 94.6437) (-16.0053, 94.7398) knots 0 0 0 0 0.074032 0.14217 0.14217 0.14217 0.14217
  spline S346 degree 3 poles (-13.4127, 94.6441) (-13.6133, 94.5758) (-14.0097, 94.4408) (-14.428, 94.4202) (-14.6347, 94.41) knots 0 0 0 0 0.0632 0.124959 0.124959 0.124959 0.124959
  spline S347 degree 3 poles (-12.4916, 95.1859) (-12.6177, 95.0833) (-12.8968, 94.8563) (-13.23, 94.7193) (-13.4127, 94.6441) knots 0 0 0 0 0.048493 0.107374 0.107374 0.107374 0.107374
  line L233 (-12.4916, 95.1859) -> (-12.4916, 97.182)
  line L234 (-12.4916, 97.182) -> (-14.6723, 97.182)
  line L235 (-14.6723, 97.182) -> (-14.6723, 96.3377)
  line L236 (-14.6723, 96.3377) -> (-13.5136, 96.3377)
  line L237 (-10.6083, 94.4954) -> (-10.6083, 97.763)
  line L238 (-10.6083, 97.763) -> (-8.5883, 94.4954)
  line L239 (-8.5883, 94.4954) -> (-7.5731, 94.4954)
  line L240 (-7.5731, 94.4954) -> (-7.5731, 99.5062)
  line L241 (-7.5731, 99.5062) -> (-8.5131, 99.5062)
  line L242 (-8.5131, 99.5062) -> (-8.5131, 96.16)
  line L243 (-8.5131, 96.16) -> (-10.5639, 99.5062)
  line L244 (-10.5639, 99.5062) -> (-11.5482, 99.5062)
  line L245 (-11.5482, 99.5062) -> (-11.5482, 94.4954)
  line L246 (-11.5482, 94.4954) -> (-10.6083, 94.4954)
  line L247 (-6.5067, 94.4954) -> (-4.6029, 94.4954)
  spline S348 degree 3 poles (-3.7074, 94.6014) (-3.8373, 94.5706) (-4.1315, 94.5009) (-4.434, 94.4974) (-4.6029, 94.4954) knots 0 0 0 0 0.039934 0.090419 0.090419 0.090419 0.090419
  spline S349 degree 3 poles (-2.9965, 95.0013) (-3.0962, 94.9193) (-3.3091, 94.7439) (-3.5691, 94.6509) (-3.7074, 94.6014) knots 0 0 0 0 0.038436 0.082116 0.082116 0.082116 0.082116
  spline S350 degree 3 poles (-2.4599, 95.8866) (-2.5264, 95.7158) (-2.6536, 95.389) (-2.8857, 95.1266) (-2.9965, 95.0013) knots 0 0 0 0 0.054482 0.104246 0.104246 0.104246 0.104246
  spline S351 degree 3 poles (-2.3061, 96.953) (-2.3105, 96.7597) (-2.3189, 96.3978) (-2.4151, 96.0491) (-2.4599, 95.8866) knots 0 0 0 0 0.057721 0.108107 0.108107 0.108107 0.108107
  spline S352 degree 3 poles (-2.4701, 98.1373) (-2.4224, 97.9595) (-2.3182, 97.572) (-2.3103, 97.1704) (-2.3061, 96.953) knots 0 0 0 0 0.055013 0.119956 0.119956 0.119956 0.119956
  spline S353 degree 3 poles (-2.9486, 98.9491) (-2.8494, 98.8303) (-2.6454, 98.5861) (-2.5296, 98.2896) (-2.4701, 98.1373) knots 0 0 0 0 0.046108 0.094787 0.094787 0.094787 0.094787
  spline S354 degree 3 poles (-3.704, 99.4105) (-3.5624, 99.3589) (-3.2796, 99.2558) (-3.0588, 99.0512) (-2.9486, 98.9491) knots 0 0 0 0 0.044725 0.089312 0.089312 0.089312 0.089312
  spline S355 degree 3 poles (-4.6576, 99.5062) (-4.4731, 99.5052) (-4.1519, 99.5035) (-3.8377, 99.4382) (-3.704, 99.4105) knots 0 0 0 0 0.055167 0.096048 0.096048 0.096048 0.096048
  line L248 (-4.6576, 99.5062) -> (-6.5067, 99.5062)
  line L249 (-6.5067, 99.5062) -> (-6.5067, 94.4954)
  spline S356 degree 3 poles (-4.2099, 98.6107) (-4.3143, 98.6245) (-4.5897, 98.6608) (-4.8678, 98.6594) (-5.0404, 98.6585) knots 0 0 0 0 0.031564 0.083275 0.083275 0.083275 0.083275
  spline S357 degree 3 poles (-3.7416, 98.3748) (-3.8088, 98.4286) (-3.9482, 98.54) (-4.1206, 98.5866) (-4.2099, 98.6107) knots 0 0 0 0 0.02553 0.052932 0.052932 0.052932 0.052932
  spline S358 degree 3 poles (-3.4545, 97.8895) (-3.4898, 97.9852) (-3.556, 98.1648) (-3.6825, 98.308) (-3.7416, 98.3748) knots 0 0 0 0 0.030297 0.056827 0.056827 0.056827 0.056827
  spline S359 degree 3 poles (-3.352, 96.9974) (-3.3532, 97.1695) (-3.3554, 97.4709) (-3.4247, 97.7638) (-3.4545, 97.8895) knots 0 0 0 0 0.051419 0.090046 0.090046 0.090046 0.090046
  spline S360 degree 3 poles (-3.4545, 96.0797) (-3.4247, 96.2118) (-3.3566, 96.5136) (-3.3536, 96.8233) (-3.352, 96.9974) knots 0 0 0 0 0.040513 0.092572 0.092572 0.092572 0.092572
  spline S361 degree 3 poles (-3.7194, 95.596) (-3.6662, 95.6585) (-3.5449, 95.801) (-3.487, 95.9795) (-3.4545, 96.0797) knots 0 0 0 0 0.024396 0.055616 0.055616 0.055616 0.055616
  spline S362 degree 3 poles (-4.1278, 95.3875) (-4.0504, 95.4106) (-3.9013, 95.455) (-3.7785, 95.5503) (-3.7194, 95.596) knots 0 0 0 0 0.023993 0.046213 0.046213 0.046213 0.046213
  spline S363 degree 3 poles (-4.7397, 95.3397) (-4.6177, 95.3397) (-4.4123, 95.3396) (-4.21, 95.3737) (-4.1278, 95.3875) knots 0 0 0 0 0.036506 0.061461 0.061461 0.061461 0.061461
  line L250 (-4.7397, 95.3397) -> (-5.495, 95.3397)
  line L251 (-5.495, 95.3397) -> (-5.495, 98.6585)
  line L252 (-5.495, 98.6585) -> (-5.0404, 98.6585)
  line L253 (65.4454, 131.2301) -> (65.4454, 132.5323)
  line L254 (65.4454, 132.5323) -> (66.7613, 132.5323)
  line L255 (66.7613, 132.5323) -> (66.7613, 133.4312)
  line L256 (66.7613, 133.4312) -> (65.4454, 133.4312)
  line L257 (65.4454, 133.4312) -> (65.4454, 134.7335)
  line L258 (65.4454, 134.7335) -> (64.5704, 134.7335)
  line L259 (64.5704, 134.7335) -> (64.5704, 133.4312)
  line L260 (64.5704, 133.4312) -> (63.2579, 133.4312)
  line L261 (63.2579, 133.4312) -> (63.2579, 132.5323)
  line L262 (63.2579, 132.5323) -> (64.5704, 132.5323)
  line L263 (64.5704, 132.5323) -> (64.5704, 131.2301)
  line L264 (64.5704, 131.2301) -> (65.4454, 131.2301)
  spline S364 degree 3 poles (60.6192, 130.42) (60.3308, 130.4304) (59.8036, 130.4493) (59.3605, 130.7314) (59.1597, 130.8592) knots 0 0 0 0 0.084711 0.154875 0.154875 0.154875 0.154875
  spline S365 degree 3 poles (61.7095, 130.6029) (61.5471, 130.5496) (61.1933, 130.4337) (60.8207, 130.4248) (60.6192, 130.42) knots 0 0 0 0 0.051011 0.111086 0.111086 0.111086 0.111086
  spline S366 degree 3 poles (62.3863, 131.1617) (62.2971, 131.0439) (62.1157, 130.8044) (61.8464, 130.6708) (61.7095, 130.6029) knots 0 0 0 0 0.043681 0.088839 0.088839 0.088839 0.088839
  spline S367 degree 3 poles (62.6255, 131.9683) (62.6152, 131.8265) (62.5944, 131.5402) (62.4561, 131.2886) (62.3863, 131.1617) knots 0 0 0 0 0.042126 0.085024 0.085024 0.085024 0.085024
  spline S368 degree 3 poles (62.4256, 132.7664) (62.4839, 132.6482) (62.6077, 132.397) (62.6194, 132.1167) (62.6255, 131.9683) knots 0 0 0 0 0.039093 0.083085 0.083085 0.083085 0.083085
  spline S369 degree 3 poles (61.8719, 133.2757) (61.9829, 133.2087) (62.2021, 133.0764) (62.3518, 132.8688) (62.4256, 132.7664) knots 0 0 0 0 0.038473 0.075924 0.075924 0.075924 0.075924
  spline S370 degree 3 poles (60.7798, 133.6363) (60.9963, 133.5843) (61.3707, 133.4945) (61.7232, 133.3406) (61.8719, 133.2757) knots 0 0 0 0 0.066618 0.115197 0.115197 0.115197 0.115197
  spline S371 degree 3 poles (59.8501, 133.9713) (59.958, 133.9126) (60.2497, 133.7541) (60.5749, 133.6818) (60.7798, 133.6363) knots 0 0 0 0 0.036685 0.099222 0.099222 0.099222 0.099222
  spline S372 degree 3 poles (59.6998, 134.2755) (59.7067, 134.2178) (59.7211, 134.099) (59.8063, 134.0147) (59.8501, 133.9713) knots 0 0 0 0 0.016915 0.034837 0.034837 0.034837 0.034837
  spline S373 degree 3 poles (59.8604, 134.5865) (59.8135, 134.5447) (59.7203, 134.4614) (59.7066, 134.3372) (59.6998, 134.2755) knots 0 0 0 0 0.018159 0.036131 0.036131 0.036131 0.036131
  spline S374 degree 3 poles (60.5508, 134.7677) (60.4168, 134.7634) (60.172, 134.7557) (59.9575, 134.6392) (59.8604, 134.5865) knots 0 0 0 0 0.039567 0.07226 0.07226 0.07226 0.07226
  spline S375 degree 3 poles (61.1917, 134.5985) (61.1047, 134.6476) (60.9068, 134.7594) (60.6786, 134.7647) (60.5508, 134.7677) knots 0 0 0 0 0.029564 0.067187 0.067187 0.067187 0.067187
  spline S376 degree 3 poles (61.4703, 134.043) (61.4466, 134.1591) (61.4035, 134.3704) (61.2575, 134.5276) (61.1917, 134.5985) knots 0 0 0 0 0.034732 0.063204 0.063204 0.063204 0.063204
  line L265 (61.4703, 134.043) -> (62.482, 134.0875)
  spline S377 degree 3 poles (61.9813, 135.1915) (62.1214, 135.0393) (62.409, 134.7268) (62.4573, 134.3042) (62.482, 134.0875) knots 0 0 0 0 0.060438 0.124056 0.124056 0.124056 0.124056
  spline S378 degree 3 poles (60.5611, 135.6051) (60.8448, 135.5967) (61.3566, 135.5816) (61.7887, 135.3117) (61.9813, 135.1915) knots 0 0 0 0 0.083316 0.150278 0.150278 0.150278 0.150278
  spline S379 degree 3 poles (59.575, 135.4307) (59.7239, 135.4815) (60.0433, 135.5904) (60.3809, 135.6) (60.5611, 135.6051) knots 0 0 0 0 0.046932 0.100643 0.100643 0.100643 0.100643
  spline S380 degree 3 poles (58.9495, 134.9232) (59.0317, 135.0284) (59.2012, 135.2453) (59.448, 135.3677) (59.575, 135.4307) knots 0 0 0 0 0.039537 0.081472 0.081472 0.081472 0.081472
  spline S381 degree 3 poles (58.7325, 134.2071) (58.7419, 134.3332) (58.7609, 134.588) (58.8862, 134.8107) (58.9495, 134.9232) knots 0 0 0 0 0.037438 0.075643 0.075643 0.075643 0.075643
  spline S382 degree 3 poles (59.1939, 133.1988) (59.0593, 133.343) (58.7933, 133.6281) (58.7526, 134.0156) (58.7325, 134.2071) knots 0 0 0 0 0.057473 0.113615 0.113615 0.113615 0.113615
  spline S383 degree 3 poles (60.3355, 132.7032) (60.0981, 132.7635) (59.6896, 132.8673) (59.3402, 133.1009) (59.1939, 133.1988) knots 0 0 0 0 0.072771 0.125248 0.125248 0.125248 0.125248
  spline S384 degree 3 poles (61.1456, 132.4845) (61.0486, 132.5135) (60.7806, 132.5939) (60.5089, 132.6606) (60.3355, 132.7032) knots 0 0 0 0 0.030365 0.083918 0.083918 0.083918 0.083918
  spline S385 degree 3 poles (61.5096, 132.2674) (61.4637, 132.3092) (61.3574, 132.4059) (61.2223, 132.456) (61.1456, 132.4845) knots 0 0 0 0 0.018463 0.042727 0.042727 0.042727 0.042727
  spline S386 degree 3 poles (61.6138, 131.9649) (61.6099, 132.0214) (61.6023, 132.1317) (61.54, 132.2229) (61.5096, 132.2674) knots 0 0 0 0 0.016654 0.032515 0.032515 0.032515 0.032515
  spline S387 degree 3 poles (61.366, 131.4813) (61.4382, 131.5509) (61.5766, 131.6843) (61.6018, 131.8742) (61.6138, 131.9649) knots 0 0 0 0 0.02913 0.055793 0.055793 0.055793 0.055793
  spline S388 degree 3 poles (60.6294, 131.2745) (60.7763, 131.2785) (61.0404, 131.2858) (61.2659, 131.4212) (61.366, 131.4813) knots 0 0 0 0 0.043164 0.077652 0.077652 0.077652 0.077652
  spline S389 degree 3 poles (59.8963, 131.5069) (59.9995, 131.4392) (60.2214, 131.2937) (60.4872, 131.2812) (60.6294, 131.2745) knots 0 0 0 0 0.036365 0.078171 0.078171 0.078171 0.078171
  spline S390 degree 3 poles (59.5357, 132.2349) (59.568, 132.0852) (59.6273, 131.8111) (59.8123, 131.6019) (59.8963, 131.5069) knots 0 0 0 0 0.045039 0.082457 0.082457 0.082457 0.082457
  line L266 (59.5357, 132.2349) -> (58.5513, 132.1392)
  spline S391 degree 3 poles (59.1597, 130.8592) (59.0063, 131.0303) (58.6785, 131.3957) (58.5955, 131.8811) (58.5513, 132.1392) knots 0 0 0 0 0.067573 0.144312 0.144312 0.144312 0.144312
  line L267 (55.1504, 130.5089) -> (55.1504, 132.399)
  line L268 (55.1504, 132.399) -> (55.8101, 132.399)
  spline S392 degree 3 poles (56.8594, 132.4708) (56.7118, 132.45) (56.3639, 132.4009) (56.0125, 132.3997) (55.8101, 132.399) knots 0 0 0 0 0.044674 0.105284 0.105284 0.105284 0.105284
  spline S393 degree 3 poles (57.3841, 132.7083) (57.2994, 132.654) (57.1361, 132.549) (56.9494, 132.4962) (56.8594, 132.4708) knots 0 0 0 0 0.029989 0.057875 0.057875 0.057875 0.057875
  spline S394 degree 3 poles (57.8096, 133.2022) (57.7515, 133.1041) (57.639, 132.914) (57.4672, 132.7754) (57.3841, 132.7083) knots 0 0 0 0 0.033903 0.065663 0.065663 0.065663 0.065663
  spline S395 degree 3 poles (57.9771, 133.9781) (57.9722, 133.8345) (57.963, 133.5654) (57.8584, 133.3177) (57.8096, 133.2022) knots 0 0 0 0 0.042674 0.079973 0.079973 0.079973 0.079973
  spline S396 degree 3 poles (57.6866, 134.9539) (57.7712, 134.8134) (57.9516, 134.5139) (57.9683, 134.1639) (57.9771, 133.9781) knots 0 0 0 0 0.048456 0.103242 0.103242 0.103242 0.103242
  spline S397 degree 3 poles (56.9654, 135.4444) (57.104, 135.3947) (57.3863, 135.2933) (57.5853, 135.0684) (57.6866, 134.9539) knots 0 0 0 0 0.043425 0.08848 0.08848 0.08848 0.08848
  spline S398 degree 3 poles (55.7623, 135.5196) (56.0169, 135.5215) (56.4201, 135.5246) (56.8186, 135.466) (56.9654, 135.4444) knots 0 0 0 0 0.076244 0.120695 0.120695 0.120695 0.120695
  line L269 (55.7623, 135.5196) -> (54.1387, 135.5196)
  line L270 (54.1387, 135.5196) -> (54.1387, 130.5089)
  line L271 (54.1387, 130.5089) -> (55.1504, 130.5089)
  spline S399 degree 3 poles (56.3672, 134.6378) (56.2764, 134.6476) (56.0346, 134.6738) (55.7912, 134.6727) (55.6392, 134.672) knots 0 0 0 0 0.027379 0.072931 0.072931 0.072931 0.072931
  spline S400 degree 3 poles (56.774, 134.4156) (56.7164, 134.4694) (56.5999, 134.5782) (56.4454, 134.6178) (56.3672, 134.6378) knots 0 0 0 0 0.023234 0.047014 0.047014 0.047014 0.047014
  spline S401 degree 3 poles (56.9346, 133.9644) (56.929, 134.0504) (56.918, 134.2163) (56.8208, 134.3508) (56.774, 134.4156) knots 0 0 0 0 0.025272 0.048763 0.048763 0.048763 0.048763
  spline S402 degree 3 poles (56.8201, 133.5748) (56.8535, 133.6337) (56.922, 133.7546) (56.9303, 133.8934) (56.9346, 133.9644) knots 0 0 0 0 0.020048 0.041093 0.041093 0.041093 0.041093
  spline S403 degree 3 poles (56.504, 133.3287) (56.5672, 133.3581) (56.6915, 133.4159) (56.7778, 133.5224) (56.8201, 133.5748) knots 0 0 0 0 0.02062 0.040539 0.040539 0.040539 0.040539
  spline S404 degree 3 poles (55.7042, 133.2501) (55.8714, 133.2487) (56.1413, 133.2466) (56.404, 133.3061) (56.504, 133.3287) knots 0 0 0 0 0.049941 0.080592 0.080592 0.080592 0.080592
  line L272 (55.7042, 133.2501) -> (55.1504, 133.2501)
  line L273 (55.1504, 133.2501) -> (55.1504, 134.672)
  line L274 (55.1504, 134.672) -> (55.6392, 134.672)
  line L275 (63.5148, 112.4954) -> (65.4186, 112.4954)
  spline S405 degree 3 poles (66.3141, 112.6014) (66.1842, 112.5706) (65.89, 112.5009) (65.5875, 112.4974) (65.4186, 112.4954) knots 0 0 0 0 0.039934 0.090419 0.090419 0.090419 0.090419
  spline S406 degree 3 poles (67.025, 113.0013) (66.9253, 112.9193) (66.7124, 112.7439) (66.4524, 112.6509) (66.3141, 112.6014) knots 0 0 0 0 0.038436 0.082116 0.082116 0.082116 0.082116
  spline S407 degree 3 poles (67.5616, 113.8866) (67.4951, 113.7158) (67.3679, 113.389) (67.1358, 113.1266) (67.025, 113.0013) knots 0 0 0 0 0.054482 0.104246 0.104246 0.104246 0.104246
  spline S408 degree 3 poles (67.7154, 114.953) (67.711, 114.7597) (67.7026, 114.3978) (67.6064, 114.0491) (67.5616, 113.8866) knots 0 0 0 0 0.057721 0.108107 0.108107 0.108107 0.108107
  spline S409 degree 3 poles (67.5514, 116.1373) (67.5991, 115.9595) (67.7033, 115.572) (67.7112, 115.1704) (67.7154, 114.953) knots 0 0 0 0 0.055013 0.119956 0.119956 0.119956 0.119956
  spline S410 degree 3 poles (67.0729, 116.9491) (67.1721, 116.8303) (67.3761, 116.5861) (67.4919, 116.2896) (67.5514, 116.1373) knots 0 0 0 0 0.046108 0.094787 0.094787 0.094787 0.094787
  spline S411 degree 3 poles (66.3175, 117.4105) (66.4591, 117.3589) (66.7419, 117.2558) (66.9627, 117.0512) (67.0729, 116.9491) knots 0 0 0 0 0.044725 0.089312 0.089312 0.089312 0.089312
  spline S412 degree 3 poles (65.3639, 117.5062) (65.5484, 117.5052) (65.8696, 117.5035) (66.1838, 117.4382) (66.3175, 117.4105) knots 0 0 0 0 0.055167 0.096048 0.096048 0.096048 0.096048
  line L276 (65.3639, 117.5062) -> (63.5148, 117.5062)
  line L277 (63.5148, 117.5062) -> (63.5148, 112.4954)
  spline S413 degree 3 poles (65.8116, 116.6107) (65.7072, 116.6245) (65.4318, 116.6608) (65.1537, 116.6594) (64.9811, 116.6585) knots 0 0 0 0 0.031564 0.083275 0.083275 0.083275 0.083275
  spline S414 degree 3 poles (66.2799, 116.3748) (66.2127, 116.4286) (66.0733, 116.54) (65.9009, 116.5866) (65.8116, 116.6107) knots 0 0 0 0 0.02553 0.052932 0.052932 0.052932 0.052932
  spline S415 degree 3 poles (66.567, 115.8895) (66.5317, 115.9852) (66.4655, 116.1648) (66.339, 116.308) (66.2799, 116.3748) knots 0 0 0 0 0.030297 0.056827 0.056827 0.056827 0.056827
  spline S416 degree 3 poles (66.6695, 114.9974) (66.6683, 115.1695) (66.6661, 115.4709) (66.5968, 115.7638) (66.567, 115.8895) knots 0 0 0 0 0.051419 0.090046 0.090046 0.090046 0.090046
  spline S417 degree 3 poles (66.567, 114.0797) (66.5968, 114.2118) (66.6649, 114.5136) (66.6679, 114.8233) (66.6695, 114.9974) knots 0 0 0 0 0.040513 0.092572 0.092572 0.092572 0.092572
  spline S418 degree 3 poles (66.3021, 113.596) (66.3553, 113.6585) (66.4766, 113.801) (66.5345, 113.9795) (66.567, 114.0797) knots 0 0 0 0 0.024396 0.055616 0.055616 0.055616 0.055616
  spline S419 degree 3 poles (65.8937, 113.3875) (65.9711, 113.4106) (66.1202, 113.455) (66.243, 113.5503) (66.3021, 113.596) knots 0 0 0 0 0.023993 0.046213 0.046213 0.046213 0.046213
  spline S420 degree 3 poles (65.2819, 113.3397) (65.4038, 113.3397) (65.6092, 113.3396) (65.8115, 113.3737) (65.8937, 113.3875) knots 0 0 0 0 0.036506 0.061461 0.061461 0.061461 0.061461
  line L278 (65.2819, 113.3397) -> (64.5265, 113.3397)
  line L279 (64.5265, 113.3397) -> (64.5265, 116.6585)
  line L280 (64.5265, 116.6585) -> (64.9811, 116.6585)
  line L281 (59.4132, 112.4954) -> (59.4132, 115.763)
  line L282 (59.4132, 115.763) -> (61.4332, 112.4954)
  line L283 (61.4332, 112.4954) -> (62.4484, 112.4954)
  line L284 (62.4484, 112.4954) -> (62.4484, 117.5062)
  line L285 (62.4484, 117.5062) -> (61.5084, 117.5062)
  line L286 (61.5084, 117.5062) -> (61.5084, 114.16)
  line L287 (61.5084, 114.16) -> (59.4576, 117.5062)
  line L288 (59.4576, 117.5062) -> (58.4733, 117.5062)
  line L289 (58.4733, 117.5062) -> (58.4733, 112.4954)
  line L290 (58.4733, 112.4954) -> (59.4132, 112.4954)
  line L291 (56.5079, 114.3377) -> (56.5079, 113.702)
  spline S421 degree 3 poles (55.9593, 113.3995) (56.0603, 113.4419) (56.254, 113.5233) (56.4257, 113.6441) (56.5079, 113.702) knots 0 0 0 0 0.032744 0.062808 0.062808 0.062808 0.062808
  spline S422 degree 3 poles (55.3219, 113.2747) (55.4289, 113.2803) (55.6473, 113.2917) (55.854, 113.3631) (55.9593, 113.3995) knots 0 0 0 0 0.031982 0.065241 0.065241 0.065241 0.065241
  spline S423 degree 3 poles (54.2828, 113.7208) (54.4274, 113.5907) (54.7229, 113.3249) (55.1194, 113.2917) (55.3219, 113.2747) knots 0 0 0 0 0.056717 0.115883 0.115883 0.115883 0.115883
  spline S424 degree 3 poles (53.8863, 115.0589) (53.8943, 114.7908) (53.9087, 114.3072) (54.1675, 113.9015) (54.2828, 113.7208) knots 0 0 0 0 0.078685 0.141874 0.141874 0.141874 0.141874
  spline S425 degree 3 poles (54.2777, 116.3065) (54.1639, 116.1378) (53.9109, 115.763) (53.895, 115.3088) (53.8863, 115.0589) knots 0 0 0 0 0.059895 0.133098 0.133098 0.133098 0.133098
  spline S426 degree 3 poles (55.3321, 116.7269) (55.1254, 116.7124) (54.7279, 116.6846) (54.4237, 116.429) (54.2777, 116.3065) knots 0 0 0 0 0.060436 0.116147 0.116147 0.116147 0.116147
  spline S427 degree 3 poles (56.0619, 116.5133) (55.955, 116.5755) (55.7299, 116.7067) (55.4691, 116.72) (55.3321, 116.7269) knots 0 0 0 0 0.036554 0.077026 0.077026 0.077026 0.077026
  spline S428 degree 3 poles (56.4601, 115.9305) (56.4178, 116.0465) (56.3346, 116.2748) (56.1518, 116.4346) (56.0619, 116.5133) knots 0 0 0 0 0.036378 0.071607 0.071607 0.071607 0.071607
  line L292 (56.4601, 115.9305) -> (57.465, 116.1185)
  spline S429 degree 3 poles (56.7899, 117.2003) (56.9497, 117.055) (57.2761, 116.7583) (57.4011, 116.3347) (57.465, 116.1185) knots 0 0 0 0 0.063491 0.129715 0.129715 0.129715 0.129715
  spline S430 degree 3 poles (55.3321, 117.5916) (55.6158, 117.5825) (56.1341, 117.5657) (56.5856, 117.3142) (56.7899, 117.2003) knots 0 0 0 0 0.083673 0.152883 0.152883 0.152883 0.152883
  spline S431 degree 3 poles (54.1324, 117.3421) (54.3105, 117.4148) (54.6944, 117.5715) (55.1096, 117.5846) (55.3321, 117.5916) knots 0 0 0 0 0.057235 0.123411 0.123411 0.123411 0.123411
  spline S432 degree 3 poles (53.172, 116.409) (53.2948, 116.6004) (53.5423, 116.986) (53.9348, 117.2228) (54.1324, 117.3421) knots 0 0 0 0 0.067249 0.13551 0.13551 0.13551 0.13551
  spline S433 degree 3 poles (52.8439, 115.0179) (52.8557, 115.268) (52.8785, 115.7525) (53.0763, 116.195) (53.172, 116.409) knots 0 0 0 0 0.074367 0.144055 0.144055 0.144055 0.144055
  spline S434 degree 3 poles (53.1378, 113.6832) (53.0521, 113.894) (52.878, 114.322) (52.8554, 114.7836) (52.8439, 115.0179) knots 0 0 0 0 0.067732 0.137548 0.137548 0.137548 0.137548
  spline S435 degree 3 poles (54.0162, 112.7398) (53.8333, 112.862) (53.4662, 113.1071) (53.2475, 113.4907) (53.1378, 113.6832) knots 0 0 0 0 0.065007 0.130489 0.130489 0.130489 0.130489
  spline S436 degree 3 poles (55.3868, 112.41) (55.1376, 112.4213) (54.659, 112.443) (54.2245, 112.6437) (54.0162, 112.7398) knots 0 0 0 0 0.074032 0.14217 0.14217 0.14217 0.14217
  spline S437 degree 3 poles (56.6088, 112.6441) (56.4082, 112.5758) (56.0118, 112.4408) (55.5935, 112.4202) (55.3868, 112.41) knots 0 0 0 0 0.0632 0.124959 0.124959 0.124959 0.124959
  spline S438 degree 3 poles (57.5299, 113.1859) (57.4038, 113.0833) (57.1247, 112.8563) (56.7915, 112.7193) (56.6088, 112.6441) knots 0 0 0 0 0.048493 0.107374 0.107374 0.107374 0.107374
  line L293 (57.5299, 113.1859) -> (57.5299, 115.182)
  line L294 (57.5299, 115.182) -> (55.3492, 115.182)
  line L295 (55.3492, 115.182) -> (55.3492, 114.3377)
  line L296 (55.3492, 114.3377) -> (56.5079, 114.3377)
  line L297 (60.5284, 90.8475) -> (59.4567, 86.8475)
  line L298 (59.4567, 86.8475) -> (61.2438, 86.8475)
  line L299 (61.2438, 86.8475) -> (60.44, 83.8475)
  line L300 (60.44, 83.8475) -> (63.7964, 87.8475)
  line L301 (63.7964, 87.8475) -> (61.2964, 87.8475)
  line L302 (61.2964, 87.8475) -> (63.0284, 90.8475)
  line L303 (63.0284, 90.8475) -> (60.5284, 90.8475)